Autodesk Inventor part; units mm, degrees
(part 4 of 5)
  line L786 (-10.0052, -6.7941) -> (-10.0052, -6.9319)
  line L787 (-10.0052, -6.9319) -> (-11.0441, -6.9319)
  spline S867 degree 2 poles (-11.0441, -6.9319) (-11.0441, -7.1928) (-10.7816, -7.47) (-10.5482, -7.47) knots 0 0 0 1 2 2 2
  spline S868 degree 2 poles (-10.5482, -7.47) (-10.4655, -7.47) (-10.3051, -7.4327) (-10.2402, -7.4035) knots 0 0 0 1 2 2 2
  spline S869 degree 2 poles (-10.2402, -7.4035) (-10.1722, -7.3711) (-10.0782, -7.3144) (-10.0474, -7.2884) knots 0 0 0 1 2 2 2
  line L788 (-10.0474, -7.2884) -> (-10.0328, -7.2884)
  line L789 (-10.0328, -7.2884) -> (-10.0328, -7.564)
  spline S870 degree 2 poles (-10.0328, -7.564) (-10.0765, -7.5818) (-10.2094, -7.6337) (-10.2613, -7.6482) knots 0 0 0 1 2 2 2
  spline S871 degree 2 poles (-10.2613, -7.6482) (-10.3342, -7.6693) (-10.4542, -7.6904) (-10.5449, -7.6904) knots 0 0 0 1 2 2 2
  spline S872 degree 2 poles (-10.2516, -6.739) (-10.2548, -6.6369) (-10.297, -6.4878) (-10.3375, -6.4376) knots 0 0 0 1 2 2 2
  spline S873 degree 2 poles (-10.3375, -6.4376) (-10.3812, -6.3808) (-10.519, -6.3209) (-10.6211, -6.3209) knots 0 0 0 1 2 2 2
  spline S874 degree 2 poles (-10.6211, -6.3209) (-10.7216, -6.3209) (-10.8626, -6.3808) (-10.921, -6.4392) knots 0 0 0 1 2 2 2
  spline S875 degree 2 poles (-10.921, -6.4392) (-10.9777, -6.4991) (-11.036, -6.6434) (-11.0441, -6.739) knots 0 0 0 1 2 2 2
  line L790 (-11.0441, -6.739) -> (-10.2516, -6.739)
  line L791 (-9.4915, -7.6564) -> (-9.7443, -7.6564)
  line L792 (-9.7443, -7.6564) -> (-9.7443, -5.5672)
  line L793 (-9.7443, -5.5672) -> (-9.4915, -5.5672)
  line L794 (-9.4915, -5.5672) -> (-9.4915, -7.6564)
  spline S876 degree 2 poles (-8.4688, -7.6904) (-8.8286, -7.6904) (-9.224, -7.2868) (-9.224, -6.914) knots 0 0 0 1 2 2 2
  spline S877 degree 2 poles (-9.224, -6.914) (-9.224, -6.5478) (-8.8399, -6.1134) (-8.5304, -6.1134) knots 0 0 0 1 2 2 2
  spline S878 degree 2 poles (-8.5304, -6.1134) (-8.391, -6.1134) (-8.1754, -6.1944) (-8.096, -6.2803) knots 0 0 0 1 2 2 2
  spline S879 degree 2 poles (-8.096, -6.2803) (-8.015, -6.3662) (-7.9291, -6.6142) (-7.9291, -6.7941) knots 0 0 0 1 2 2 2
  line L795 (-7.9291, -6.7941) -> (-7.9291, -6.9319)
  line L796 (-7.9291, -6.9319) -> (-8.968, -6.9319)
  spline S880 degree 2 poles (-8.968, -6.9319) (-8.968, -7.1928) (-8.7054, -7.47) (-8.472, -7.47) knots 0 0 0 1 2 2 2
  spline S881 degree 2 poles (-8.472, -7.47) (-8.3893, -7.47) (-8.2289, -7.4327) (-8.1641, -7.4035) knots 0 0 0 1 2 2 2
  spline S882 degree 2 poles (-8.1641, -7.4035) (-8.096, -7.3711) (-8.002, -7.3144) (-7.9712, -7.2884) knots 0 0 0 1 2 2 2
  line L797 (-7.9712, -7.2884) -> (-7.9566, -7.2884)
  line L798 (-7.9566, -7.2884) -> (-7.9566, -7.564)
  spline S883 degree 2 poles (-7.9566, -7.564) (-8.0004, -7.5818) (-8.1333, -7.6337) (-8.1851, -7.6482) knots 0 0 0 1 2 2 2
  spline S884 degree 2 poles (-8.1851, -7.6482) (-8.2581, -7.6693) (-8.378, -7.6904) (-8.4688, -7.6904) knots 0 0 0 1 2 2 2
  spline S885 degree 2 poles (-8.1754, -6.739) (-8.1787, -6.6369) (-8.2208, -6.4878) (-8.2613, -6.4376) knots 0 0 0 1 2 2 2
  spline S886 degree 2 poles (-8.2613, -6.4376) (-8.3051, -6.3808) (-8.4428, -6.3209) (-8.5449, -6.3209) knots 0 0 0 1 2 2 2
  spline S887 degree 2 poles (-8.5449, -6.3209) (-8.6454, -6.3209) (-8.7864, -6.3808) (-8.8448, -6.4392) knots 0 0 0 1 2 2 2
  spline S888 degree 2 poles (-8.8448, -6.4392) (-8.9015, -6.4991) (-8.9599, -6.6434) (-8.968, -6.739) knots 0 0 0 1 2 2 2
  line L799 (-8.968, -6.739) -> (-8.1754, -6.739)
  spline S889 degree 2 poles (-28.3034, -10.0611) (-28.3034, -10.2556) (-28.5822, -10.5328) (-28.7767, -10.5328) knots 0 0 0 1 2 2 2
  spline S890 degree 2 poles (-28.7767, -10.5328) (-28.9712, -10.5328) (-29.2483, -10.2556) (-29.2483, -10.0611) knots 0 0 0 1 2 2 2
  spline S891 degree 2 poles (-29.2483, -10.0611) (-29.2483, -9.8666) (-28.9712, -9.5895) (-28.7767, -9.5895) knots 0 0 0 1 2 2 2
  spline S892 degree 2 poles (-28.7767, -9.5895) (-28.5822, -9.5895) (-28.3034, -9.8666) (-28.3034, -10.0611) knots 0 0 0 1 2 2 2
  spline S893 degree 2 poles (-22.6406, -10.985) (-22.8577, -10.985) (-23.1624, -10.8942) (-23.297, -10.8294) knots 0 0 0 1 2 2 2
  line L800 (-23.297, -10.8294) -> (-23.297, -10.4955)
  line L801 (-23.297, -10.4955) -> (-23.2775, -10.4955)
  spline S894 degree 2 poles (-23.2775, -10.4955) (-23.1462, -10.6187) (-22.814, -10.7548) (-22.66, -10.7548) knots 0 0 0 1 2 2 2
  spline S895 degree 2 poles (-22.66, -10.7548) (-22.4396, -10.7548) (-22.2143, -10.5717) (-22.2143, -10.4209) knots 0 0 0 1 2 2 2
  spline S896 degree 2 poles (-22.2143, -10.4209) (-22.2143, -10.301) (-22.3326, -10.1519) (-22.4607, -10.1146) knots 0 0 0 1 2 2 2
  spline S897 degree 2 poles (-22.4607, -10.1146) (-22.553, -10.0887) (-22.707, -10.053) (-22.8221, -10.0239) knots 0 0 0 1 2 2 2
  spline S898 degree 2 poles (-22.8221, -10.0239) (-22.9258, -9.9963) (-23.0895, -9.9136) (-23.1527, -9.8472) knots 0 0 0 1 2 2 2
  spline S899 degree 2 poles (-23.1527, -9.8472) (-23.2143, -9.7807) (-23.2824, -9.6025) (-23.2824, -9.4858) knots 0 0 0 1 2 2 2
  spline S900 degree 2 poles (-23.2824, -9.4858) (-23.2824, -9.2427) (-22.9031, -8.9136) (-22.6098, -8.9136) knots 0 0 0 1 2 2 2
  spline S901 degree 2 poles (-22.6098, -8.9136) (-22.4412, -8.9136) (-22.143, -8.9801) (-22.015, -9.0433) knots 0 0 0 1 2 2 2
  line L802 (-22.015, -9.0433) -> (-22.015, -9.361)
  line L803 (-22.015, -9.361) -> (-22.0344, -9.361)
  spline S902 degree 2 poles (-22.0344, -9.361) (-22.13, -9.2734) (-22.4282, -9.1438) (-22.5919, -9.1438) knots 0 0 0 1 2 2 2
  spline S903 degree 2 poles (-22.5919, -9.1438) (-22.7767, -9.1438) (-23.0052, -9.3172) (-23.0052, -9.4582) knots 0 0 0 1 2 2 2
  spline S904 degree 2 poles (-23.0052, -9.4582) (-23.0052, -9.5846) (-22.8707, -9.7354) (-22.7443, -9.7694) knots 0 0 0 1 2 2 2
  spline S905 degree 2 poles (-22.7443, -9.7694) (-22.66, -9.7921) (-22.4153, -9.8504) (-22.3342, -9.8747) knots 0 0 0 1 2 2 2
  spline S906 degree 2 poles (-22.3342, -9.8747) (-22.1284, -9.938) (-21.9372, -10.1924) (-21.9372, -10.3788) knots 0 0 0 1 2 2 2
  spline S907 degree 2 poles (-21.9372, -10.3788) (-21.9372, -10.4971) (-22.0328, -10.724) (-22.1187, -10.8034) knots 0 0 0 1 2 2 2
  spline S908 degree 2 poles (-22.1187, -10.8034) (-22.2143, -10.891) (-22.4574, -10.985) (-22.6406, -10.985) knots 0 0 0 1 2 2 2
  spline S909 degree 2 poles (-20.4526, -10.1989) (-20.4526, -10.5781) (-20.8172, -10.9914) (-21.1219, -10.9914) knots 0 0 0 1 2 2 2
  spline S910 degree 2 poles (-21.1219, -10.9914) (-21.4347, -10.9914) (-21.7929, -10.5652) (-21.7929, -10.1989) knots 0 0 0 1 2 2 2
  spline S911 degree 2 poles (-21.7929, -10.1989) (-21.7929, -9.8229) (-21.4234, -9.4063) (-21.1219, -9.4063) knots 0 0 0 1 2 2 2
  spline S912 degree 2 poles (-21.1219, -9.4063) (-20.8172, -9.4063) (-20.4526, -9.8213) (-20.4526, -10.1989) knots 0 0 0 1 2 2 2
  spline S913 degree 2 poles (-20.7135, -10.1989) (-20.7135, -9.9072) (-20.9258, -9.6235) (-21.1219, -9.6235) knots 0 0 0 1 2 2 2
  spline S914 degree 2 poles (-21.1219, -9.6235) (-21.318, -9.6235) (-21.532, -9.9072) (-21.532, -10.1989) knots 0 0 0 1 2 2 2
  spline S915 degree 2 poles (-21.532, -10.1989) (-21.532, -10.4825) (-21.318, -10.7743) (-21.1219, -10.7743) knots 0 0 0 1 2 2 2
  spline S916 degree 2 poles (-21.1219, -10.7743) (-20.9274, -10.7743) (-20.7135, -10.4874) (-20.7135, -10.1989) knots 0 0 0 1 2 2 2
  spline S917 degree 2 poles (-19.5968, -10.9833) (-19.7524, -10.9833) (-20.0101, -10.8877) (-20.1025, -10.7905) knots 0 0 0 1 2 2 2
  spline S918 degree 2 poles (-20.1025, -10.7905) (-20.1949, -10.6948) (-20.297, -10.3999) (-20.297, -10.2021) knots 0 0 0 1 2 2 2
  spline S919 degree 2 poles (-20.297, -10.2021) (-20.297, -10.0044) (-20.1916, -9.7159) (-20.1025, -9.6187) knots 0 0 0 1 2 2 2
  spline S920 degree 2 poles (-20.1025, -9.6187) (-20.0133, -9.5198) (-19.7492, -9.4145) (-19.5968, -9.4145) knots 0 0 0 1 2 2 2
  spline S921 degree 2 poles (-19.5968, -9.4145) (-19.4736, -9.4145) (-19.2435, -9.4841) (-19.1543, -9.5295) knots 0 0 0 1 2 2 2
  line L804 (-19.1543, -9.5295) -> (-19.1543, -9.8132)
  line L805 (-19.1543, -9.8132) -> (-19.1689, -9.8132)
  spline S922 degree 2 poles (-19.1689, -9.8132) (-19.1965, -9.7905) (-19.2808, -9.7321) (-19.3407, -9.7013) knots 0 0 0 1 2 2 2
  spline S923 degree 2 poles (-19.3407, -9.7013) (-19.3942, -9.6754) (-19.5368, -9.6349) (-19.6017, -9.6349) knots 0 0 0 1 2 2 2
  spline S924 degree 2 poles (-19.6017, -9.6349) (-19.7978, -9.6349) (-20.036, -9.9315) (-20.036, -10.2021) knots 0 0 0 1 2 2 2
  spline S925 degree 2 poles (-20.036, -10.2021) (-20.036, -10.4663) (-19.8059, -10.7629) (-19.6017, -10.7629) knots 0 0 0 1 2 2 2
  spline S926 degree 2 poles (-19.6017, -10.7629) (-19.4785, -10.7629) (-19.2548, -10.6608) (-19.1689, -10.5814) knots 0 0 0 1 2 2 2
  line L806 (-19.1689, -10.5814) -> (-19.1543, -10.5814)
  line L807 (-19.1543, -10.5814) -> (-19.1543, -10.865)
  spline S927 degree 2 poles (-19.1543, -10.865) (-19.1916, -10.8828) (-19.3051, -10.9331) (-19.3505, -10.9444) knots 0 0 0 1 2 2 2
  spline S928 degree 2 poles (-19.3505, -10.9444) (-19.4153, -10.9639) (-19.5174, -10.9833) (-19.5968, -10.9833) knots 0 0 0 1 2 2 2
  spline S929 degree 2 poles (-18.3278, -10.9833) (-18.4834, -10.9833) (-18.7411, -10.8877) (-18.8334, -10.7905) knots 0 0 0 1 2 2 2
  spline S930 degree 2 poles (-18.8334, -10.7905) (-18.9258, -10.6948) (-19.0279, -10.3999) (-19.0279, -10.2021) knots 0 0 0 1 2 2 2
  spline S931 degree 2 poles (-19.0279, -10.2021) (-19.0279, -10.0044) (-18.9226, -9.7159) (-18.8334, -9.6187) knots 0 0 0 1 2 2 2
  spline S932 degree 2 poles (-18.8334, -9.6187) (-18.7443, -9.5198) (-18.4801, -9.4145) (-18.3278, -9.4145) knots 0 0 0 1 2 2 2
  spline S933 degree 2 poles (-18.3278, -9.4145) (-18.2046, -9.4145) (-17.9744, -9.4841) (-17.8853, -9.5295) knots 0 0 0 1 2 2 2
  line L808 (-17.8853, -9.5295) -> (-17.8853, -9.8132)
  line L809 (-17.8853, -9.8132) -> (-17.8999, -9.8132)
  spline S934 degree 2 poles (-17.8999, -9.8132) (-17.9274, -9.7905) (-18.0117, -9.7321) (-18.0717, -9.7013) knots 0 0 0 1 2 2 2
  spline S935 degree 2 poles (-18.0717, -9.7013) (-18.1252, -9.6754) (-18.2678, -9.6349) (-18.3326, -9.6349) knots 0 0 0 1 2 2 2
  spline S936 degree 2 poles (-18.3326, -9.6349) (-18.5287, -9.6349) (-18.767, -9.9315) (-18.767, -10.2021) knots 0 0 0 1 2 2 2
  spline S937 degree 2 poles (-18.767, -10.2021) (-18.767, -10.4663) (-18.5368, -10.7629) (-18.3326, -10.7629) knots 0 0 0 1 2 2 2
  spline S938 degree 2 poles (-18.3326, -10.7629) (-18.2094, -10.7629) (-17.9858, -10.6608) (-17.8999, -10.5814) knots 0 0 0 1 2 2 2
  line L810 (-17.8999, -10.5814) -> (-17.8853, -10.5814)
  line L811 (-17.8853, -10.5814) -> (-17.8853, -10.865)
  spline S939 degree 2 poles (-17.8853, -10.865) (-17.9226, -10.8828) (-18.036, -10.9331) (-18.0814, -10.9444) knots 0 0 0 1 2 2 2
  spline S940 degree 2 poles (-18.0814, -10.9444) (-18.1462, -10.9639) (-18.2483, -10.9833) (-18.3278, -10.9833) knots 0 0 0 1 2 2 2
  line L812 (-17.3975, -10.9493) -> (-17.6503, -10.9493)
  line L813 (-17.6503, -10.9493) -> (-17.6503, -9.4485)
  line L814 (-17.6503, -9.4485) -> (-17.3975, -9.4485)
  line L815 (-17.3975, -9.4485) -> (-17.3975, -10.9493)
  line L816 (-17.3796, -9.1989) -> (-17.6665, -9.1989)
  line L817 (-17.6665, -9.1989) -> (-17.6665, -8.9363)
  line L818 (-17.6665, -8.9363) -> (-17.3796, -8.9363)
  line L819 (-17.3796, -8.9363) -> (-17.3796, -9.1989)
  spline S941 degree 2 poles (-15.7929, -10.1989) (-15.7929, -10.5781) (-16.1576, -10.9914) (-16.4623, -10.9914) knots 0 0 0 1 2 2 2
  spline S942 degree 2 poles (-16.4623, -10.9914) (-16.7751, -10.9914) (-17.1333, -10.5652) (-17.1333, -10.1989) knots 0 0 0 1 2 2 2
  spline S943 degree 2 poles (-17.1333, -10.1989) (-17.1333, -9.8229) (-16.7637, -9.4063) (-16.4623, -9.4063) knots 0 0 0 1 2 2 2
  spline S944 degree 2 poles (-16.4623, -9.4063) (-16.1576, -9.4063) (-15.7929, -9.8213) (-15.7929, -10.1989) knots 0 0 0 1 2 2 2
  spline S945 degree 2 poles (-16.0539, -10.1989) (-16.0539, -9.9072) (-16.2662, -9.6235) (-16.4623, -9.6235) knots 0 0 0 1 2 2 2
  spline S946 degree 2 poles (-16.4623, -9.6235) (-16.6584, -9.6235) (-16.8723, -9.9072) (-16.8723, -10.1989) knots 0 0 0 1 2 2 2
  spline S947 degree 2 poles (-16.8723, -10.1989) (-16.8723, -10.4825) (-16.6584, -10.7743) (-16.4623, -10.7743) knots 0 0 0 1 2 2 2
  spline S948 degree 2 poles (-16.4623, -10.7743) (-16.2678, -10.7743) (-16.0539, -10.4874) (-16.0539, -10.1989) knots 0 0 0 1 2 2 2
  line L820 (-13.4963, -10.9493) -> (-14.6552, -10.9493)
  line L821 (-14.6552, -10.9493) -> (-14.6552, -8.9493)
  line L822 (-14.6552, -8.9493) -> (-14.3893, -8.9493)
  line L823 (-14.3893, -8.9493) -> (-14.3893, -10.7127)
  line L824 (-14.3893, -10.7127) -> (-13.4963, -10.7127)
  line L825 (-13.4963, -10.7127) -> (-13.4963, -10.9493)
  spline S949 degree 2 poles (-12.6552, -10.9833) (-13.015, -10.9833) (-13.4104, -10.5798) (-13.4104, -10.207) knots 0 0 0 1 2 2 2
  spline S950 degree 2 poles (-13.4104, -10.207) (-13.4104, -9.8407) (-13.0263, -9.4063) (-12.7167, -9.4063) knots 0 0 0 1 2 2 2
  spline S951 degree 2 poles (-12.7167, -9.4063) (-12.5774, -9.4063) (-12.3618, -9.4874) (-12.2824, -9.5733) knots 0 0 0 1 2 2 2
  spline S952 degree 2 poles (-12.2824, -9.5733) (-12.2013, -9.6592) (-12.1154, -9.9072) (-12.1154, -10.0871) knots 0 0 0 1 2 2 2
  line L826 (-12.1154, -10.0871) -> (-12.1154, -10.2248)
  line L827 (-12.1154, -10.2248) -> (-13.1543, -10.2248)
  spline S953 degree 2 poles (-13.1543, -10.2248) (-13.1543, -10.4858) (-12.8918, -10.7629) (-12.6584, -10.7629) knots 0 0 0 1 2 2 2
  spline S954 degree 2 poles (-12.6584, -10.7629) (-12.5757, -10.7629) (-12.4153, -10.7256) (-12.3505, -10.6965) knots 0 0 0 1 2 2 2
  spline S955 degree 2 poles (-12.3505, -10.6965) (-12.2824, -10.664) (-12.1884, -10.6073) (-12.1576, -10.5814) knots 0 0 0 1 2 2 2
  line L828 (-12.1576, -10.5814) -> (-12.143, -10.5814)
  line L829 (-12.143, -10.5814) -> (-12.143, -10.8569)
  spline S956 degree 2 poles (-12.143, -10.8569) (-12.1868, -10.8747) (-12.3197, -10.9266) (-12.3715, -10.9412) knots 0 0 0 1 2 2 2
  spline S957 degree 2 poles (-12.3715, -10.9412) (-12.4445, -10.9623) (-12.5644, -10.9833) (-12.6552, -10.9833) knots 0 0 0 1 2 2 2
  spline S958 degree 2 poles (-12.3618, -10.032) (-12.365, -9.9298) (-12.4072, -9.7807) (-12.4477, -9.7305) knots 0 0 0 1 2 2 2
  spline S959 degree 2 poles (-12.4477, -9.7305) (-12.4915, -9.6738) (-12.6292, -9.6138) (-12.7313, -9.6138) knots 0 0 0 1 2 2 2
  spline S960 degree 2 poles (-12.7313, -9.6138) (-12.8318, -9.6138) (-12.9728, -9.6738) (-13.0312, -9.7321) knots 0 0 0 1 2 2 2
  spline S961 degree 2 poles (-13.0312, -9.7321) (-13.0879, -9.7921) (-13.1462, -9.9363) (-13.1543, -10.032) knots 0 0 0 1 2 2 2
  line L830 (-13.1543, -10.032) -> (-12.3618, -10.032)
  spline S962 degree 2 poles (-10.626, -10.1989) (-10.626, -10.5781) (-10.9906, -10.9914) (-11.2953, -10.9914) knots 0 0 0 1 2 2 2
  spline S963 degree 2 poles (-11.2953, -10.9914) (-11.6081, -10.9914) (-11.9663, -10.5652) (-11.9663, -10.1989) knots 0 0 0 1 2 2 2
  spline S964 degree 2 poles (-11.9663, -10.1989) (-11.9663, -9.8229) (-11.5968, -9.4063) (-11.2953, -9.4063) knots 0 0 0 1 2 2 2
  spline S965 degree 2 poles (-11.2953, -9.4063) (-10.9906, -9.4063) (-10.626, -9.8213) (-10.626, -10.1989) knots 0 0 0 1 2 2 2
  spline S966 degree 2 poles (-10.8869, -10.1989) (-10.8869, -9.9072) (-11.0992, -9.6235) (-11.2953, -9.6235) knots 0 0 0 1 2 2 2
  spline S967 degree 2 poles (-11.2953, -9.6235) (-11.4915, -9.6235) (-11.7054, -9.9072) (-11.7054, -10.1989) knots 0 0 0 1 2 2 2
  spline S968 degree 2 poles (-11.7054, -10.1989) (-11.7054, -10.4825) (-11.4915, -10.7743) (-11.2953, -10.7743) knots 0 0 0 1 2 2 2
  spline S969 degree 2 poles (-11.2953, -10.7743) (-11.1009, -10.7743) (-10.8869, -10.4874) (-10.8869, -10.1989) knots 0 0 0 1 2 2 2
  line L831 (-9.1884, -10.9493) -> (-9.4412, -10.9493)
  line L832 (-9.4412, -10.9493) -> (-9.4412, -10.0935)
  spline S970 degree 2 poles (-9.4412, -10.0935) (-9.4412, -9.9898) (-9.4607, -9.8115) (-9.4898, -9.758) knots 0 0 0 1 2 2 2
  spline S971 degree 2 poles (-9.4898, -9.758) (-9.5206, -9.7013) (-9.6308, -9.6462) (-9.7248, -9.6462) knots 0 0 0 1 2 2 2
  spline S972 degree 2 poles (-9.7248, -9.6462) (-9.8188, -9.6462) (-10.0182, -9.7467) (-10.1138, -9.8277) knots 0 0 0 1 2 2 2
  line L833 (-10.1138, -9.8277) -> (-10.1138, -10.9493)
  line L834 (-10.1138, -10.9493) -> (-10.3667, -10.9493)
  line L835 (-10.3667, -10.9493) -> (-10.3667, -9.4485)
  line L836 (-10.3667, -9.4485) -> (-10.1138, -9.4485)
  line L837 (-10.1138, -9.4485) -> (-10.1138, -9.6154)
  spline S973 degree 2 poles (-10.1138, -9.6154) (-10.0004, -9.5133) (-9.7816, -9.4063) (-9.6584, -9.4063) knots 0 0 0 1 2 2 2
  spline S974 degree 2 poles (-9.6584, -9.4063) (-9.438, -9.4063) (-9.1884, -9.6981) (-9.1884, -9.9752) knots 0 0 0 1 2 2 2
  line L838 (-9.1884, -9.9752) -> (-9.1884, -10.9493)
  spline S975 degree 2 poles (-7.9971, -10.7905) (-8.0279, -10.8132) (-8.1317, -10.8942) (-8.1803, -10.9185) knots 0 0 0 1 2 2 2
  spline S976 degree 2 poles (-8.1803, -10.9185) (-8.2467, -10.9542) (-8.3715, -10.9914) (-8.485, -10.9914) knots 0 0 0 1 2 2 2
  spline S977 degree 2 poles (-8.485, -10.9914) (-8.5774, -10.9914) (-8.7443, -10.9217) (-8.8075, -10.8585) knots 0 0 0 1 2 2 2
  spline S978 degree 2 poles (-8.8075, -10.8585) (-8.8675, -10.7969) (-8.9404, -10.6154) (-8.9404, -10.5149) knots 0 0 0 1 2 2 2
  spline S979 degree 2 poles (-8.9404, -10.5149) (-8.9404, -10.3593) (-8.8091, -10.1389) (-8.6665, -10.0757) knots 0 0 0 1 2 2 2
  spline S980 degree 2 poles (-8.6665, -10.0757) (-8.5401, -10.0174) (-8.1965, -9.9736) (-7.9971, -9.9623) knots 0 0 0 1 2 2 2
  line L839 (-7.9971, -9.9623) -> (-7.9971, -9.9136)
  spline S981 degree 2 poles (-7.9971, -9.9136) (-7.9971, -9.8261) (-8.0506, -9.7175) (-8.0992, -9.6867) knots 0 0 0 1 2 2 2
  spline S982 degree 2 poles (-8.0992, -9.6867) (-8.1479, -9.6559) (-8.2872, -9.6365) (-8.3618, -9.6365) knots 0 0 0 1 2 2 2
  spline S983 degree 2 poles (-8.3618, -9.6365) (-8.4493, -9.6365) (-8.6859, -9.6884) (-8.8043, -9.7386) knots 0 0 0 1 2 2 2
  line L840 (-8.8043, -9.7386) -> (-8.8188, -9.7386)
  line L841 (-8.8188, -9.7386) -> (-8.8188, -9.4809)
  spline S984 degree 2 poles (-8.8188, -9.4809) (-8.7492, -9.4615) (-8.4882, -9.4128) (-8.3602, -9.4128) knots 0 0 0 1 2 2 2
  spline S985 degree 2 poles (-8.3602, -9.4128) (-8.2046, -9.4128) (-7.9923, -9.4615) (-7.908, -9.5247) knots 0 0 0 1 2 2 2
  spline S986 degree 2 poles (-7.908, -9.5247) (-7.8253, -9.5863) (-7.7443, -9.7824) (-7.7443, -9.9234) knots 0 0 0 1 2 2 2
  line L842 (-7.7443, -9.9234) -> (-7.7443, -10.9493)
  line L843 (-7.7443, -10.9493) -> (-7.9971, -10.9493)
  line L844 (-7.9971, -10.9493) -> (-7.9971, -10.7905)
  line L845 (-7.9971, -10.5798) -> (-7.9971, -10.1632)
  spline S987 degree 2 poles (-7.9971, -10.1632) (-8.0879, -10.1713) (-8.3618, -10.1989) (-8.4477, -10.2248) knots 0 0 0 1 2 2 2
  spline S988 degree 2 poles (-8.4477, -10.2248) (-8.5482, -10.2556) (-8.6795, -10.3837) (-8.6795, -10.4971) knots 0 0 0 1 2 2 2
  spline S989 degree 2 poles (-8.6795, -10.4971) (-8.6795, -10.6268) (-8.5336, -10.758) (-8.3942, -10.758) knots 0 0 0 1 2 2 2
  spline S990 degree 2 poles (-8.3942, -10.758) (-8.2759, -10.758) (-8.0814, -10.6559) (-7.9971, -10.5798) knots 0 0 0 1 2 2 2
  line L846 (-6.5936, -9.7192) -> (-6.6065, -9.7192)
  spline S991 degree 2 poles (-6.6065, -9.7192) (-6.6357, -9.711) (-6.6989, -9.7078) (-6.7427, -9.7078) knots 0 0 0 1 2 2 2
  spline S992 degree 2 poles (-6.7427, -9.7078) (-6.8448, -9.7078) (-7.0458, -9.7969) (-7.1365, -9.8845) knots 0 0 0 1 2 2 2
  line L847 (-7.1365, -9.8845) -> (-7.1365, -10.9493)
  line L848 (-7.1365, -10.9493) -> (-7.3893, -10.9493)
  line L849 (-7.3893, -10.9493) -> (-7.3893, -9.4485)
  line L850 (-7.3893, -9.4485) -> (-7.1365, -9.4485)
  line L851 (-7.1365, -9.4485) -> (-7.1365, -9.6722)
  spline S993 degree 2 poles (-7.1365, -9.6722) (-6.9987, -9.549) (-6.7929, -9.4485) (-6.6957, -9.4485) knots 0 0 0 1 2 2 2
  spline S994 degree 2 poles (-6.6957, -9.4485) (-6.6568, -9.4485) (-6.6179, -9.4517) (-6.5936, -9.4566) knots 0 0 0 1 2 2 2
  line L852 (-6.5936, -9.4566) -> (-6.5936, -9.7192)
  line L853 (-5.2435, -10.9493) -> (-5.4963, -10.9493)
  line L854 (-5.4963, -10.9493) -> (-5.4963, -10.7969)
  spline S995 degree 2 poles (-5.4963, -10.7969) (-5.5547, -10.8456) (-5.6406, -10.9104) (-5.6989, -10.938) knots 0 0 0 1 2 2 2
  spline S996 degree 2 poles (-5.6989, -10.938) (-5.7524, -10.9639) (-5.8675, -10.9914) (-5.9436, -10.9914) knots 0 0 0 1 2 2 2
  spline S997 degree 2 poles (-5.9436, -10.9914) (-6.0668, -10.9914) (-6.2743, -10.8893) (-6.3472, -10.7905) knots 0 0 0 1 2 2 2
  spline S998 degree 2 poles (-6.3472, -10.7905) (-6.4201, -10.6916) (-6.5012, -10.3999) (-6.5012, -10.2102) knots 0 0 0 1 2 2 2
  spline S999 degree 2 poles (-6.5012, -10.2102) (-6.5012, -10.0125) (-6.3991, -9.724) (-6.3099, -9.6154) knots 0 0 0 1 2 2 2
  spline S1000 degree 2 poles (-6.3099, -9.6154) (-6.2273, -9.5182) (-5.9955, -9.4063) (-5.8675, -9.4063) knots 0 0 0 1 2 2 2
  spline S1001 degree 2 poles (-5.8675, -9.4063) (-5.7556, -9.4063) (-5.5887, -9.4566) (-5.4963, -9.5085) knots 0 0 0 1 2 2 2
  line L855 (-5.4963, -9.5085) -> (-5.4963, -8.8602)
  line L856 (-5.4963, -8.8602) -> (-5.2435, -8.8602)
  line L857 (-5.2435, -8.8602) -> (-5.2435, -10.9493)
  line L858 (-5.4963, -10.5846) -> (-5.4963, -9.7175)
  spline S1002 degree 2 poles (-5.4963, -9.7175) (-5.5903, -9.6722) (-5.7394, -9.6381) (-5.8253, -9.6381) knots 0 0 0 1 2 2 2
  spline S1003 degree 2 poles (-5.8253, -9.6381) (-6.0198, -9.6381) (-6.2402, -9.9298) (-6.2402, -10.2054) knots 0 0 0 1 2 2 2
  spline S1004 degree 2 poles (-6.2402, -10.2054) (-6.2402, -10.4712) (-6.0717, -10.7516) (-5.8853, -10.7516) knots 0 0 0 1 2 2 2
  spline S1005 degree 2 poles (-5.8853, -10.7516) (-5.7864, -10.7516) (-5.5855, -10.6608) (-5.4963, -10.5846) knots 0 0 0 1 2 2 2
  spline S1006 degree 2 poles (-3.6438, -10.1989) (-3.6438, -10.5781) (-4.0085, -10.9914) (-4.3132, -10.9914) knots 0 0 0 1 2 2 2
  spline S1007 degree 2 poles (-4.3132, -10.9914) (-4.626, -10.9914) (-4.9842, -10.5652) (-4.9842, -10.1989) knots 0 0 0 1 2 2 2
  spline S1008 degree 2 poles (-4.9842, -10.1989) (-4.9842, -9.8229) (-4.6146, -9.4063) (-4.3132, -9.4063) knots 0 0 0 1 2 2 2
  spline S1009 degree 2 poles (-4.3132, -9.4063) (-4.0085, -9.4063) (-3.6438, -9.8213) (-3.6438, -10.1989) knots 0 0 0 1 2 2 2
  spline S1010 degree 2 poles (-3.9047, -10.1989) (-3.9047, -9.9072) (-4.1171, -9.6235) (-4.3132, -9.6235) knots 0 0 0 1 2 2 2
  spline S1011 degree 2 poles (-4.3132, -9.6235) (-4.5093, -9.6235) (-4.7232, -9.9072) (-4.7232, -10.1989) knots 0 0 0 1 2 2 2
  spline S1012 degree 2 poles (-4.7232, -10.1989) (-4.7232, -10.4825) (-4.5093, -10.7743) (-4.3132, -10.7743) knots 0 0 0 1 2 2 2
  spline S1013 degree 2 poles (-4.3132, -10.7743) (-4.1187, -10.7743) (-3.9047, -10.4874) (-3.9047, -10.1989) knots 0 0 0 1 2 2 2
  point P0 (0, 0)
  constraints: 48 end point, 12 horizontal, 12 vertical, 26 other
extrude "Estrusione2" cut sketch "Schizzo2" against normal blind 1 contours S0 S1 L32 L33 L34 L35 L36 S2 S3 | L40 S8 S9 L41 L42 L43 L44 L45 S10 S11 L46 | S12 S13 S14 S15 | S20 S21 S22 S23 L47 S24 S25 S26 S27 S28 L48 L49 L50 S29 S30 L51 L52 | S35 S36 S37 S38 L54 L55 S39 S40 S41 L56 L57 S42 S43 | S48 L59 L60 L61 L62 L63 L64 L65 L66 L67 L68 L69 S49 S50 S51 L70 L71 S52 | S53 L72 L73 L74 L75 L76 L77 L78 L79 L80 L81 L82 S54 S55 S56 L83 L84 S57 | S58 S59 S60 S61 | L85 L86 S66 S67 S68 S69 S70 S71 S72 L87 L88 L89 | L91 L92 L93 L94 | L95 L96 L97 L98 | L99 S77 S78 S79 S80 L100 L101 L102 S81 S82 S83 L103 L104 L105 L106 L107 S84 S85 S86 S87 S88 L108 L109 | S89 S90 S91 S92 L110 L111 S93 S94 S95 L112 L113 S96 S97 | S102 S103 S104 S105 S106 L115 L116 S107 S108 S109 S110 S111 L117 L118 S112 S113 | S114 S115 S116 S117 S118 L119 L120 S119 S120 S121 S122 S123 L121 L122 S124 S125 | S126 S127 S128 S129 S130 S131 L123 S132 S133 S134 L124 L125 S135 S136 S137 L126 L127 L128 | L130 L131 S142 S143 S144 L132 L133 L134 L135 L136 S145 S146 L137 | L138 L139 L140 L141 | L142 L143 L144 L145 | S147 S148 S149 S150 S151 L146 L147 S152 S153 S154 S155 S156 L148 L149 S157 S158 | S159 S160 S161 S162 S163 S164 L150 S165 S166 S167 L151 L152 S168 S169 S170 L153 L154 L155 | L157 L158 S175 S176 S177 S178 S179 S180 S181 L159 L160 L161 | S186 S187 S188 S189 L163 L164 S190 S191 S192 L165 L166 S193 S194 | L168 L169 L170 L171 | L172 L173 L174 L175 | S199 S200 S201 S202 L176 L177 S203 S204 S205 L178 L179 S206 S207 | L181 L182 L183 L184 L185 L186 L187 | L188 L189 L190 L191 | L192 L193 L194 L195 | S212 S213 L196 L197 L198 L199 L200 S214 S215 | L202 S220 S221 L203 L204 L205 L206 L207 S222 S223 L208 | S224 S225 S226 S227 S228 S229 L209 S230 S231 S232 L210 L211 S233 S234 S235 L212 L213 L214 | L216 L217 L218 L219 L220 L221 L222 L223 L224 L225 | L226 L227 L228 L229 | L230 L231 L232 L233 | S240 S241 S242 S243 | L234 L235 S248 S249 S250 L236 L237 L238 L239 L240 S251 S252 L241 | L242 L243 L244 L245 | L246 L247 L248 L249 | L250 L251 S253 S254 S255 S256 S257 S258 L252 L253 S259 S260 S261 S262 S263 L254 L255 | S264 S265 S266 S267 | L256 L257 L258 L259 L260 L261 S276 L262 L263 L264 L265 | S277 S278 S279 S280 S281 S282 S283 L266 L267 S284 S285 S286 S287 S288 | L268 L269 L270 L271 | L272 L273 S296 S297 S298 S299 S300 S301 L274 L275 S302 S303 S304 S305 S306 L276 L277 | S307 S308 S309 S310 | S319 S320 L278 L279 L280 S321 S322 S323 L281 S324 | S333 S334 S335 S336 S337 S338 L288 S339 S340 S341 L289 L290 S342 S343 S344 L291 L292 L293 | L295 L296 S349 S350 S351 L297 L298 L299 L300 L301 S352 S353 L302 | S354 S355 S356 S357 S358 L303 L304 S359 S360 S361 S362 S363 L305 L306 S364 S365 | S366 S367 S368 S369 | L307 L308 S374 S375 S376 S377 S378 S379 S380 L309 L310 L311 | L313 L314 L315 L316 | L317 L318 L319 L320 | S385 S386 L321 L322 L323 L324 L325 S387 S388 | L327 S393 S394 L328 L329 L330 L331 L332 S395 S396 L333 | S397 S398 S399 S400 | L334 L335 L336 L337 L338 L339 L340 | S405 S406 S407 S408 S409 S410 L341 S411 S412 S413 L342 L343 S414 S415 S416 L344 L345 L346 | S421 S422 L348 L349 L350 L351 L352 S423 S424 | S429 S430 S431 S432 L354 L355 S433 S434 S435 L356 L357 S436 S437 | L359 S442 S443 L360 L361 L362 L363 L364 S444 S445 L365 | L366 S446 S447 S448 S449 L367 L368 L369 S450 S451 S452 L370 L371 L372 L373 L374 S453 S454 S455 S456 S457 L375 L376 | S458 S459 S460 S461 | S466 L377 L378 L379 L380 L381 L382 L383 L384 L385 L386 L387 S467 S468 S469 L388 L389 S470 | S471 S472 S473 S474 | L390 S479 S480 L391 L392 L393 L394 L395 S481 S482 L396 | S483 S484 S485 S486 L397 L398 S487 S488 S489 L399 L400 S490 S491 | S496 S497 L402 L403 L404 S498 S499 | S504 S505 S506 S507 S508 S509 L408 L409 S510 S511 S512 S513 S514 S515 S516 S517 L410 L411 S518 S519 | L412 L413 L414 L415 L416 L417 L418 L419 | S520 S521 S522 S523 S524 L423 L424 S525 S526 S527 S528 S529 L425 L426 S530 S531 | L427 L428 S532 S533 S534 L429 L430 L431 S535 S536 S537 L432 L433 L434 | L435 S538 S539 L436 L437 L438 L439 L440 S540 S541 L441 | S542 S543 S544 S545 S546 S547 L442 S548 S549 S550 L443 L444 S551 S552 S553 L445 L446 L447 | L449 L450 S558 S559 S560 S561 S562 S563 S564 L451 L452 L453 | L455 L456 L457 L458 | L459 L460 L461 L462 | L463 L464 L465 L466 | L467 L468 L469 L470 | S569 S570 S571 S572 | L471 L472 L473 L474 L475 L476 L477 L478 | L482 L483 L484 L485 | L486 S573 S574 L487 L488 L489 L490 L491 L492 L493 L494 L495 L496 L497 S575 S576 L498 | S577 S578 S579 S580 S581 S582 L499 S583 S584 S585 L500 L501 S586 S587 S588 L502 L503 L504 | L506 L507 S593 S594 S595 L508 L509 L510 L511 L512 S596 S597 L513 | S598 S599 S600 S601 | L514 L515 L516 L517 L518 L519 L520 L521 L522 L523 L524 L525 | L526 S606 S607 S608 S609 L527 L528 L529 S610 S611 S612 L530 L531 L532 L533 L534 S613 S614 S615 S616 S617 L535 L536 | S618 S619 S620 S621 S622 S623 L537 S624 S625 S626 L538 L539 S627 S628 S629 L540 L541 L542 | L544 L545 S634 S635 S636 L546 L547 L548 L549 L550 S637 S638 L551 | L552 L553 S639 S640 S641 L554 L555 L556 S642 S643 S644 L557 L558 L559 | S645 S646 S647 S648 L560 L561 S649 S650 S651 L562 L563 S652 S653 | L565 L566 L567 L568 | S658 S659 S660 S661 L569 L570 S662 S663 S664 L571 L572 S665 S666 | S671 S672 S673 S674 | S675 S676 L574 L575 L576 S677 S678 S679 L577 S680 | S689 S690 S691 S692 S693 S694 L584 S695 S696 S697 L585 L586 S698 S699 S700 L587 L588 L589 | L591 L592 S705 S706 S707 S708 S709 S710 S711 L593 L594 L595 | S716 S717 S718 S719 S720 S721 L597 S722 S723 S724 L598 L599 S725 S726 S727 L600 L601 L602 | L604 L605 L606 L607 | S732 S733 S734 S735 S736 S737 L608 S738 S739 S740 L609 L610 S741 S742 S743 L611 L612 L613 | L615 S748 S749 S750 S751 L616 L617 L618 S752 S753 S754 L619 L620 L621 L622 L623 S755 S756 S757 S758 S759 L624 L625 | S760 S761 S762 S763 L626 L627 S764 S765 S766 L628 L629 S767 S768 | L631 L632 S773 S774 S775 L633 L634 L635 L636 L637 S776 S777 L638 | S778 L639 L640 L641 L642 L643 L644 L645 L646 L647 L648 L649 S779 S780 S781 L650 L651 S782 | L652 L653 L654 L655 | L656 L657 L658 L659 | L660 L661 L662 L663 L664 L665 L666 L667 L668 L669 | L670 L671 L672 L673 | L674 L675 L676 L677 | L678 L679 L680 L681 | L682 L683 L684 L685 | L686 L687 L688 L689 | S783 S784 L690 L691 L692 L693 L694 S785 S786 | S791 S792 L696 L697 L698 L699 L700 S793 S794 | S799 S800 S801 S802 | S807 S808 S809 S810 | L702 L703 L704 L705 L706 L707 L708 | L709 L710 L711 L712 | L713 L714 L715 L716 | S811 L717 L718 L719 L720 L721 L722 L723 L724 L725 L726 L727 S812 S813 S814 L728 L729 S815 | S816 L730 L731 L732 L733 L734 L735 L736 L737 L738 L739 L740 S817 S818 S819 L741 L742 S820 | L743 L744 L745 L746 | L747 L748 L749 L750 | S821 S822 S823 S824 S825 S826 L751 L752 S827 S828 S829 S830 S831 S832 L753 L754 L755 L756 L757 S833 S834 | S835 S836 S837 S838 S839 S840 L758 S841 S842 S843 L759 L760 S844 S845 S846 L761 L762 L763 | S851 S852 L765 L766 L767 L768 L769 S853 S854 | L771 S859 S860 L772 L773 L774 L775 L776 S861 S862 L777 | L778 L779 L780 L781 | L782 L783 L784 L785 | S863 S864 S865 S866 L786 L787 S867 S868 S869 L788 L789 S870 S871 | L791 L792 L793 L794 | S876 S877 S878 S879 L795 L796 S880 S881 S882 L797 L798 S883 S884 | S889 S890 S891 S892 | S893 L800 L801 S894 S895 S896 S897 S898 S899 S900 S901 L802 L803 S902 S903 S904 S905 S906 S907 S908 | S909 S910 S911 S912 | S917 S918 S919 S920 S921 L804 L805 S922 S923 S924 S925 S926 L806 L807 S927 S928 | S929 S930 S931 S932 S933 L808 L809 S934 S935 S936 S937 S938 L810 L811 S939 S940 | L812 L813 L814 L815 | L816 L817 L818 L819 | S941 S942 S943 S944 | L820 L821 L822 L823 L824 L825 | S949 S950 S951 S952 L826 L827 S953 S954 S955 L828 L829 S956 S957 | S962 S963 S964 S965 | L831 L832 S970 S971 S972 L833 L834 L835 L836 L837 S973 S974 L838 | S975 S976 S977 S978 S979 S980 L839 S981 S982 S983 L840 L841 S984 S985 S986 L842 L843 L844 | L846 S991 S992 L847 L848 L849 L850 L851 S993 S994 L852 | L853 L854 S995 S996 S997 S998 S999 S1000 S1001 L855 L856 L857 | S1006 S1007 S1008 S1009
sketch "Schizzo3" plane through (0, 0, 4) normal (0, 0, 1) x (1, 0, 0)
  line L0 (-31, -5) -> (-35, -5)
  line L1 (-35, -5) -> (-35, 0)
  line L2 (-35, 0) -> (-31, 0)
  line L3 (-31, 0) -> (-31, -5)
  line L4 (-35, 10) -> (-31, 10)
  line L5 (-31, 10) -> (-31, 5)
  line L6 (-31, 5) -> (-35, 5)
  line L7 (-35, 5) -> (-35, 10)
  line L8 (-31, -15) -> (-35, -15)
  line L9 (-35, -15) -> (-35, -10)
  line L10 (-35, -10) -> (-31, -10)
  line L11 (-31, -10) -> (-31, -15)
  line L12 (35, -5) -> (31, -5)
  line L13 (31, -5) -> (31, 0)
  line L14 (31, 0) -> (35, 0)
  line L15 (35, 0) -> (35, -5)
  line L16 (31, 10) -> (35, 10)
  line L17 (35, 10) -> (35, 5)
  line L18 (35, 5) -> (31, 5)
  line L19 (31, 5) -> (31, 10)
  line L20 (35, -15) -> (31, -15)
  line L21 (31, -15) -> (31, -10)
  line L22 (31, -10) -> (35, -10)
  line L23 (35, -10) -> (35, -15)
  point P0 (0, 0)
  constraints: 48 end point, 12 horizontal, 12 vertical, 24 other
extrude "Estrusione3" cut sketch "Schizzo3" against normal blind 10
sketch "Schizzo4" plane through (0, 0, 4) normal (0, 0, 1) x (1, 0, 0)
  line L0 (-31, 5) -> (-31, 10)
  line L1 (-31, 10) -> (-35, 10)
  line L2 (-35, 10) -> (-35, 12)
  arc A0 (-32, 15) -> (-35, 12) centre (-32, 12) ccw
  line L3 (-32, 15) -> (32, 15)
  arc A1 (35, 12) -> (32, 15) centre (32, 12) ccw
  line L4 (35, 12) -> (35, 10)
  line L5 (35, 10) -> (31, 10)
  line L6 (31, 10) -> (31, 5)
  line L7 (31, 5) -> (35, 5)
  line L8 (35, 5) -> (35, 0)
  line L9 (35, 0) -> (31, 0)
  line L10 (31, 0) -> (31, -5)
  line L11 (31, -5) -> (35, -5)
  line L12 (35, -5) -> (35, -10)
  line L13 (35, -10) -> (31, -10)
  line L14 (31, -10) -> (31, -15)
  line L15 (31, -15) -> (-31, -15)
  line L16 (-31, -15) -> (-31, -10)
  line L17 (-31, -10) -> (-35, -10)
  line L18 (-35, -10) -> (-35, -5)
  line L19 (-35, -5) -> (-31, -5)
  line L20 (-31, -5) -> (-31, 0)
  line L21 (-31, 0) -> (-35, 0)
  line L22 (-35, 0) -> (-35, 5)
  line L23 (-35, 5) -> (-31, 5)
  line L24 (-5.4963, -9.7175) -> (-5.4963, -10.5846)
  line L25 (-5.2435, -10.9493) -> (-5.2435, -8.8602)
  line L26 (-5.2435, -8.8602) -> (-5.4963, -8.8602)
  line L27 (-5.4963, -8.8602) -> (-5.4963, -9.5085)
  line L28 (-5.4963, -10.7969) -> (-5.4963, -10.9493)
  line L29 (-5.4963, -10.9493) -> (-5.2435, -10.9493)
  line L30 (-9.1884, -10.9493) -> (-9.1884, -9.9752)
  line L31 (-10.1138, -9.6154) -> (-10.1138, -9.4485)
  line L32 (-10.1138, -9.4485) -> (-10.3667, -9.4485)
  line L33 (-10.3667, -9.4485) -> (-10.3667, -10.9493)
  line L34 (-10.3667, -10.9493) -> (-10.1138, -10.9493)
  line L35 (-10.1138, -10.9493) -> (-10.1138, -9.8277)
  line L36 (-9.4412, -10.0935) -> (-9.4412, -10.9493)
  line L37 (-9.4412, -10.9493) -> (-9.1884, -10.9493)
  line L38 (-12.3618, -10.032) -> (-13.1543, -10.032)
  line L39 (-12.143, -10.8569) -> (-12.143, -10.5814)
  line L40 (-12.143, -10.5814) -> (-12.1576, -10.5814)
  line L41 (-13.1543, -10.2248) -> (-12.1154, -10.2248)
  line L42 (-12.1154, -10.2248) -> (-12.1154, -10.0871)
  line L43 (-17.3796, -9.1989) -> (-17.3796, -8.9363)
  line L44 (-17.3796, -8.9363) -> (-17.6665, -8.9363)
  line L45 (-17.6665, -8.9363) -> (-17.6665, -9.1989)
  line L46 (-17.6665, -9.1989) -> (-17.3796, -9.1989)
  line L47 (-17.8853, -10.865) -> (-17.8853, -10.5814)
  line L48 (-17.8853, -10.5814) -> (-17.8999, -10.5814)
  line L49 (-17.8999, -9.8132) -> (-17.8853, -9.8132)
  line L50 (-17.8853, -9.8132) -> (-17.8853, -9.5295)
  line L51 (-22.0344, -9.361) -> (-22.015, -9.361)
  line L52 (-22.015, -9.361) -> (-22.015, -9.0433)
  line L53 (-23.2775, -10.4955) -> (-23.297, -10.4955)
  line L54 (-23.297, -10.4955) -> (-23.297, -10.8294)
  line L55 (-9.4915, -7.6564) -> (-9.4915, -5.5672)
  line L56 (-9.4915, -5.5672) -> (-9.7443, -5.5672)
  line L57 (-9.7443, -5.5672) -> (-9.7443, -7.6564)
  line L58 (-9.7443, -7.6564) -> (-9.4915, -7.6564)
  line L59 (-10.2516, -6.739) -> (-11.0441, -6.739)
  line L60 (-10.0328, -7.564) -> (-10.0328, -7.2884)
  line L61 (-10.0328, -7.2884) -> (-10.0474, -7.2884)
  line L62 (-11.0441, -6.9319) -> (-10.0052, -6.9319)
  line L63 (-10.0052, -6.9319) -> (-10.0052, -6.7941)
  line L64 (-11.5676, -7.6564) -> (-11.5676, -6.1555)
  line L65 (-11.5676, -6.1555) -> (-11.8205, -6.1555)
  line L66 (-11.8205, -6.1555) -> (-11.8205, -7.6564)
  line L67 (-11.8205, -7.6564) -> (-11.5676, -7.6564)
  line L68 (-16.096, -7.5234) -> (-16.096, -6.6499)
  line L69 (-16.096, -6.6499) -> (-16.8221, -6.6499)
  line L70 (-16.8221, -6.6499) -> (-16.8221, -6.8833)
  line L71 (-16.8221, -6.8833) -> (-16.3586, -6.8833)
  line L72 (-16.3586, -6.8833) -> (-16.3586, -7.4003)
  line L73 (-16.1268, -6.1134) -> (-16.1041, -6.1134)
  line L74 (-16.1041, -6.1134) -> (-16.1041, -5.7925)
  line L75 (-18.848, -7.6564) -> (-18.848, -6.1555)
  line L76 (-18.848, -6.1555) -> (-19.1009, -6.1555)
  line L77 (-19.1009, -6.1555) -> (-19.1009, -7.6564)
  line L78 (-19.1009, -7.6564) -> (-18.848, -7.6564)
  line L79 (-20.2127, -7.6434) -> (-20.2127, -7.4165)
  line L80 (-20.2127, -7.4165) -> (-20.2273, -7.4165)
  line L81 (-20.6778, -7.0794) -> (-20.6778, -6.3646)
  line L82 (-20.6778, -6.3646) -> (-20.2127, -6.3646)
  line L83 (-20.2127, -6.3646) -> (-20.2127, -6.1555)
  line L84 (-20.2127, -6.1555) -> (-20.6778, -6.1555)
  line L85 (-20.6778, -6.1555) -> (-20.6778, -5.7244)
  line L86 (-20.6778, -5.7244) -> (-20.9307, -5.7244)
  line L87 (-20.9307, -5.7244) -> (-20.9307, -6.1555)
  line L88 (-20.9307, -6.1555) -> (-21.1009, -6.1555)
  line L89 (-21.1009, -6.1555) -> (-21.1009, -6.3646)
  line L90 (-21.1009, -6.3646) -> (-20.9307, -6.3646)
  line L91 (-20.9307, -6.3646) -> (-20.9307, -7.1961)
  line L92 (-21.318, -7.6564) -> (-21.318, -6.1555)
  line L93 (-21.318, -6.1555) -> (-21.5709, -6.1555)
  line L94 (-21.5709, -6.1555) -> (-21.5709, -7.6564)
  line L95 (-21.5709, -7.6564) -> (-21.318, -7.6564)
  line L96 (-2.3229, -4.083) -> (-2.3229, -3.2305)
  line L97 (-2.3229, -3.0198) -> (-2.3229, -2.8626)
  line L98 (-2.3229, -2.8626) -> (-2.5757, -2.8626)
  line L99 (-2.5757, -2.8626) -> (-2.5757, -4.9161)
  line L100 (-2.5757, -4.9161) -> (-2.3229, -4.9161)
  line L101 (-2.3229, -4.9161) -> (-2.3229, -4.2872)
  line L102 (-3.8432, -4.083) -> (-3.8432, -3.2305)
  line L103 (-3.8432, -3.0198) -> (-3.8432, -2.8626)
  line L104 (-3.8432, -2.8626) -> (-4.096, -2.8626)
  line L105 (-4.096, -2.8626) -> (-4.096, -4.9161)
  line L106 (-4.096, -4.9161) -> (-3.8432, -4.9161)
  line L107 (-3.8432, -4.9161) -> (-3.8432, -4.2872)
  line L108 (-4.4671, -4.3634) -> (-4.4671, -2.8626)
  line L109 (-4.4671, -2.8626) -> (-4.72, -2.8626)
  line L110 (-4.72, -2.8626) -> (-4.72, -4.3634)
  line L111 (-4.72, -4.3634) -> (-4.4671, -4.3634)
  line L112 (-5.707, -2.613) -> (-5.707, -2.3504)
  line L113 (-5.707, -2.3504) -> (-5.9939, -2.3504)
  line L114 (-5.9939, -2.3504) -> (-5.9939, -2.613)
  line L115 (-5.9939, -2.613) -> (-5.707, -2.613)
  line L116 (-6.2013, -2.6) -> (-6.2013, -2.3634)
  line L117 (-6.2013, -2.3634) -> (-7.3975, -2.3634)
  line L118 (-7.3975, -2.3634) -> (-7.3975, -4.3634)
  line L119 (-7.3975, -4.3634) -> (-7.1317, -4.3634)
  line L120 (-7.1317, -4.3634) -> (-7.1317, -3.4007)
  line L121 (-7.1317, -3.4007) -> (-6.2402, -3.4007)
  line L122 (-6.2402, -3.4007) -> (-6.2402, -3.1641)
  line L123 (-6.2402, -3.1641) -> (-7.1317, -3.1641)
  line L124 (-7.1317, -3.1641) -> (-7.1317, -2.6)
  line L125 (-7.1317, -2.6) -> (-6.2013, -2.6)
  line L126 (-8.647, -4.3634) -> (-8.647, -2.8626)
  line L127 (-8.647, -2.8626) -> (-8.8999, -2.8626)
  line L128 (-8.8999, -2.8626) -> (-8.8999, -4.3634)
  line L129 (-8.8999, -4.3634) -> (-8.647, -4.3634)
  line L130 (-10.1803, -4.3634) -> (-10.1803, -3.3893)
  line L131 (-11.1057, -3.0295) -> (-11.1057, -2.8626)
  line L132 (-11.1057, -2.8626) -> (-11.3586, -2.8626)
  line L133 (-11.3586, -2.8626) -> (-11.3586, -4.3634)
  line L134 (-11.3586, -4.3634) -> (-11.1057, -4.3634)
  line L135 (-11.1057, -4.3634) -> (-11.1057, -3.2418)
  line L136 (-10.4331, -3.5076) -> (-10.4331, -4.3634)
  line L137 (-10.4331, -4.3634) -> (-10.1803, -4.3634)
  line L138 (-11.861, -3.4461) -> (-12.6535, -3.4461)
  line L139 (-11.6422, -4.271) -> (-11.6422, -3.9955)
  line L140 (-11.6422, -3.9955) -> (-11.6568, -3.9955)
  line L141 (-12.6535, -3.6389) -> (-11.6146, -3.6389)
  line L142 (-11.6146, -3.6389) -> (-11.6146, -3.5012)
  line L143 (-16.9307, -4.3634) -> (-16.9307, -2.2743)
  line L144 (-16.9307, -2.2743) -> (-17.1835, -2.2743)
  line L145 (-17.1835, -2.2743) -> (-17.1835, -4.3634)
  line L146 (-17.1835, -4.3634) -> (-16.9307, -4.3634)
  line L147 (-17.7962, -3.5773) -> (-17.7962, -3.9939)
  line L148 (-17.7962, -4.2046) -> (-17.7962, -4.3634)
  line L149 (-17.7962, -4.3634) -> (-17.5433, -4.3634)
  line L150 (-17.5433, -4.3634) -> (-17.5433, -3.3375)
  line L151 (-18.6179, -2.895) -> (-18.6179, -3.1527)
  line L152 (-18.6179, -3.1527) -> (-18.6033, -3.1527)
  line L153 (-17.7962, -3.3277) -> (-17.7962, -3.3764)
  line L154 (-19.2516, -3.1316) -> (-19.2516, -3.9987)
  line L155 (-18.9987, -4.3634) -> (-18.9987, -2.2743)
  line L156 (-18.9987, -2.2743) -> (-19.2516, -2.2743)
  line L157 (-19.2516, -2.2743) -> (-19.2516, -2.9226)
  line L158 (-19.2516, -4.2111) -> (-19.2516, -4.3634)
  line L159 (-19.2516, -4.3634) -> (-18.9987, -4.3634)
  line L160 (-20.7605, -3.5773) -> (-20.7605, -3.9939)
  line L161 (-20.7605, -4.2046) -> (-20.7605, -4.3634)
  line L162 (-20.7605, -4.3634) -> (-20.5077, -4.3634)
  line L163 (-20.5077, -4.3634) -> (-20.5077, -3.3375)
  line L164 (-21.5822, -2.895) -> (-21.5822, -3.1527)
  line L165 (-21.5822, -3.1527) -> (-21.5676, -3.1527)
  line L166 (-20.7605, -3.3277) -> (-20.7605, -3.3764)
  line L167 (-3.3505, -0.1531) -> (-4.143, -0.1531)
  line L168 (-3.1317, -0.9781) -> (-3.1317, -0.7025)
  line L169 (-3.1317, -0.7025) -> (-3.1462, -0.7025)
  line L170 (-4.143, -0.346) -> (-3.1041, -0.346)
  line L171 (-3.1041, -0.346) -> (-3.1041, -0.2082)
  line L172 (-6.7378, -1.0705) -> (-6.7378, 0.4304)
  line L173 (-6.7378, 0.4304) -> (-6.9906, 0.4304)
  line L174 (-6.9906, 0.4304) -> (-6.9906, -0.6912)
  line L175 (-7.6633, -0.4254) -> (-7.6633, 0.4304)
  line L176 (-7.6633, 0.4304) -> (-7.9161, 0.4304)
  line L177 (-7.9161, 0.4304) -> (-7.9161, -0.5437)
  line L178 (-6.9906, -0.9051) -> (-6.9906, -1.0705)
  line L179 (-6.9906, -1.0705) -> (-6.7378, -1.0705)
  line L180 (-11.4898, -1.0705) -> (-11.237, -1.0705)
  line L181 (-11.237, -1.0705) -> (-11.237, -0.0818)
  line L182 (-12.9388, 0.265) -> (-12.9388, 0.4304)
  line L183 (-12.9388, 0.4304) -> (-13.1916, 0.4304)
  line L184 (-13.1916, 0.4304) -> (-13.1916, -1.0705)
  line L185 (-13.1916, -1.0705) -> (-12.9388, -1.0705)
  line L186 (-12.9388, -1.0705) -> (-12.9388, 0.0511)
  line L187 (-12.3407, -0.2017) -> (-12.3407, -1.0705)
  line L188 (-12.3407, -1.0705) -> (-12.0879, -1.0705)
  line L189 (-12.0879, -1.0705) -> (-12.0879, -0.0818)
  line L190 (-11.4898, -0.2017) -> (-11.4898, -1.0705)
  line L191 (-17.4412, -1.0705) -> (-17.4412, -0.0964)
  line L192 (-18.3667, 0.2634) -> (-18.3667, 0.4304)
  line L193 (-18.3667, 0.4304) -> (-18.6195, 0.4304)
  line L194 (-18.6195, 0.4304) -> (-18.6195, -1.0705)
  line L195 (-18.6195, -1.0705) -> (-18.3667, -1.0705)
  line L196 (-18.3667, -1.0705) -> (-18.3667, 0.0511)
  line L197 (-17.694, -0.2147) -> (-17.694, -1.0705)
  line L198 (-17.694, -1.0705) -> (-17.4412, -1.0705)
  line L199 (-19.2273, -0.2844) -> (-19.2273, -0.7009)
  line L200 (-19.2273, -0.9116) -> (-19.2273, -1.0705)
  line L201 (-19.2273, -1.0705) -> (-18.9744, -1.0705)
  line L202 (-18.9744, -1.0705) -> (-18.9744, -0.0445)
  line L203 (-20.049, 0.3979) -> (-20.049, 0.1402)
  line L204 (-20.049, 0.1402) -> (-20.0344, 0.1402)
  line L205 (-19.2273, -0.0348) -> (-19.2273, -0.0834)
  line L206 (-21.3099, -1.0705) -> (-21.3099, 1.0187)
  line L207 (-21.3099, 1.0187) -> (-21.5628, 1.0187)
  line L208 (-21.5628, 1.0187) -> (-21.5628, -1.0705)
  line L209 (-21.5628, -1.0705) -> (-21.3099, -1.0705)
  line L210 (-22.8902, -0.2844) -> (-22.5822, 0.6573)
  line L211 (-22.5822, 0.6573) -> (-22.2727, -0.2844)
  line L212 (-22.2727, -0.2844) -> (-22.8902, -0.2844)
  line L213 (-23.4137, -1.0705) -> (-23.1446, -1.0705)
  line L214 (-23.1446, -1.0705) -> (-22.9631, -0.5113)
  line L215 (-22.9631, -0.5113) -> (-22.1997, -0.5113)
  line L216 (-22.1997, -0.5113) -> (-22.0182, -1.0705)
  line L217 (-22.0182, -1.0705) -> (-21.7378, -1.0705)
  line L218 (-21.7378, -1.0705) -> (-22.412, 0.9295)
  line L219 (-22.412, 0.9295) -> (-22.7394, 0.9295)
  line L220 (-22.7394, 0.9295) -> (-23.4137, -1.0705)
  line L221 (-17.9987, 3.3408) -> (-17.9987, 3.7233)
  line L222 (-17.9987, 3.7233) -> (-18.3197, 3.7233)
  line L223 (-18.3197, 3.7233) -> (-18.3197, 3.3408)
  line L224 (-18.3197, 3.3408) -> (-17.9987, 3.3408)
  line L225 (-18.8156, 3.9729) -> (-18.8156, 4.2355)
  line L226 (-18.8156, 4.2355) -> (-19.1025, 4.2355)
  line L227 (-19.1025, 4.2355) -> (-19.1025, 3.9729)
  line L228 (-19.1025, 3.9729) -> (-18.8156, 3.9729)
  line L229 (-23.1106, 3.4526) -> (-23.1106, 3.7152)
  line L230 (-23.6535, 3.4996) -> (-23.6535, 3.7233)
  line L231 (-23.6535, 3.7233) -> (-23.9064, 3.7233)
  line L232 (-23.9064, 3.7233) -> (-23.9064, 2.2225)
  line L233 (-23.9064, 2.2225) -> (-23.6535, 2.2225)
  line L234 (-23.6535, 2.2225) -> (-23.6535, 3.2873)
  line L235 (-23.1235, 3.4526) -> (-23.1106, 3.4526)
  line L236 (-25.6697, 2.3068) -> (-25.6697, 2.5904)
  line L237 (-25.6697, 2.5904) -> (-25.6843, 2.5904)
  line L238 (-25.6843, 3.3586) -> (-25.6697, 3.3586)
  line L239 (-25.6697, 3.3586) -> (-25.6697, 3.6423)
  line L240 (-28.8902, 3.0086) -> (-28.5822, 3.9502)
  line L241 (-28.5822, 3.9502) -> (-28.2727, 3.0086)
  line L242 (-28.2727, 3.0086) -> (-28.8902, 3.0086)
  line L243 (-29.4137, 2.2225) -> (-29.1446, 2.2225)
  line L244 (-29.1446, 2.2225) -> (-28.9631, 2.7816)
  line L245 (-28.9631, 2.7816) -> (-28.1997, 2.7816)
  line L246 (-28.1997, 2.7816) -> (-28.0182, 2.2225)
  line L247 (-28.0182, 2.2225) -> (-27.7378, 2.2225)
  line L248 (-27.7378, 2.2225) -> (-28.412, 4.2225)
  line L249 (-28.412, 4.2225) -> (-28.7394, 4.2225)
  line L250 (-28.7394, 4.2225) -> (-29.4137, 2.2225)
  line L251 (1.5166, 6.7456) -> (1.5166, 7.0081)
  line L252 (0.9737, 6.7926) -> (0.9737, 7.0162)
  line L253 (0.9737, 7.0162) -> (0.7209, 7.0162)
  line L254 (0.7209, 7.0162) -> (0.7209, 5.5154)
  line L255 (0.7209, 5.5154) -> (0.9737, 5.5154)
  line L256 (0.9737, 5.5154) -> (0.9737, 6.5803)
  line L257 (1.5037, 6.7456) -> (1.5166, 6.7456)
  line L258 (-3.7929, 5.5154) -> (-3.5401, 5.5154)
  line L259 (-3.5401, 5.5154) -> (-3.5401, 6.5041)
  line L260 (-5.2419, 6.8509) -> (-5.2419, 7.0162)
  line L261 (-5.2419, 7.0162) -> (-5.4947, 7.0162)
  line L262 (-5.4947, 7.0162) -> (-5.4947, 5.5154)
  line L263 (-5.4947, 5.5154) -> (-5.2419, 5.5154)
  line L264 (-5.2419, 5.5154) -> (-5.2419, 6.637)
  line L265 (-4.6438, 6.3842) -> (-4.6438, 5.5154)
  line L266 (-4.6438, 5.5154) -> (-4.391, 5.5154)
  line L267 (-4.391, 5.5154) -> (-4.391, 6.5041)
  line L268 (-3.7929, 6.3842) -> (-3.7929, 5.5154)
  line L269 (-12.8075, 7.0162) -> (-13.0701, 7.0162)
  line L270 (-13.0701, 7.0162) -> (-13.4769, 5.8607)
  line L271 (-13.4769, 5.8607) -> (-13.8869, 7.0162)
  line L272 (-13.8869, 7.0162) -> (-14.1608, 7.0162)
  line L273 (-14.1608, 7.0162) -> (-13.6, 5.5154)
  line L274 (-13.6, 5.5154) -> (-13.3731, 5.5154)
  line L275 (-13.3731, 5.5154) -> (-12.8075, 7.0162)
  line L276 (-19.203, 7.2658) -> (-19.203, 7.5284)
  line L277 (-19.203, 7.5284) -> (-19.4898, 7.5284)
  line L278 (-19.4898, 7.5284) -> (-19.4898, 7.2658)
  line L279 (-19.4898, 7.2658) -> (-19.203, 7.2658)
  line L280 (-23.5806, 5.5997) -> (-23.5806, 5.8833)
  line L281 (-23.5806, 5.8833) -> (-23.5952, 5.8833)
  line L282 (-23.5952, 6.6516) -> (-23.5806, 6.6516)
  line L283 (-23.5806, 6.6516) -> (-23.5806, 6.9352)
  line L284 (-28.6308, 6.7034) -> (-28.9323, 6.7034)
  line L285 (-28.9323, 6.7034) -> (-28.9323, 7.2885)
  line L286 (-28.9323, 7.2885) -> (-28.6778, 7.2885)
  line L287 (-28.7167, 5.7423) -> (-28.9323, 5.7423)
  line L288 (-28.9323, 5.7423) -> (-28.9323, 6.4814)
  line L289 (-28.9323, 6.4814) -> (-28.6308, 6.4814)
  line L290 (-28.2159, 6.6273) -> (-28.2159, 6.637)
  line L291 (-28.6681, 7.5154) -> (-29.1981, 7.5154)
  line L292 (-29.1981, 7.5154) -> (-29.1981, 5.5154)
  line L293 (-29.1981, 5.5154) -> (-28.6244, 5.5154)
  line L294 (24.0742, 10.8975) -> (23.844, 10.8975)
  line L295 (23.844, 10.8975) -> (23.0645, 8.374)
  line L296 (23.0645, 8.374) -> (23.2914, 8.374)
  line L297 (23.2914, 8.374) -> (24.0742, 10.8975)
  line L298 (21.8732, 9.0547) -> (21.8602, 9.0547)
  line L299 (21.8602, 9.0547) -> (21.8602, 8.797)
  line L300 (18.4729, 8.8084) -> (18.4729, 9.0402)
  line L301 (18.4729, 9.0402) -> (17.4907, 9.0402)
  line L302 (17.2816, 10.7306) -> (17.2816, 10.4453)
  line L303 (17.2816, 10.4453) -> (17.2962, 10.4453)
  line L304 (17.2395, 9.092) -> (17.2395, 8.8084)
  line L305 (17.2395, 8.8084) -> (18.4729, 8.8084)
  line L306 (16.0466, 8.8084) -> (16.0466, 10.3092)
  line L307 (16.0466, 10.3092) -> (15.7938, 10.3092)
  line L308 (15.7938, 10.3092) -> (15.7938, 8.8084)
  line L309 (15.7938, 8.8084) -> (16.0466, 8.8084)
  line L310 (12.4097, 10.5588) -> (12.4097, 10.8214)
  line L311 (12.4097, 10.8214) -> (12.1228, 10.8214)
  line L312 (12.1228, 10.8214) -> (12.1228, 10.5588)
  line L313 (12.1228, 10.5588) -> (12.4097, 10.5588)
  line L314 (11.8975, 8.8084) -> (11.8975, 9.0207)
  line L315 (11.8975, 9.0207) -> (11.0953, 9.0207)
  line L316 (11.0953, 9.0207) -> (11.8829, 10.1293)
  line L317 (11.8829, 10.1293) -> (11.8829, 10.3092)
  line L318 (11.8829, 10.3092) -> (10.8278, 10.3092)
  line L319 (10.8278, 10.3092) -> (10.8278, 10.1017)
  line L320 (10.8278, 10.1017) -> (11.5799, 10.1017)
  line L321 (11.5799, 10.1017) -> (10.7954, 8.9964)
  line L322 (10.7954, 8.9964) -> (10.7954, 8.8084)
  line L323 (10.7954, 8.8084) -> (11.8975, 8.8084)
  line L324 (10.3043, 9.5944) -> (10.3043, 9.1779)
  line L325 (10.3043, 8.9672) -> (10.3043, 8.8084)
  line L326 (10.3043, 8.8084) -> (10.5572, 8.8084)
  line L327 (10.5572, 8.8084) -> (10.5572, 9.8343)
  line L328 (9.4826, 10.2768) -> (9.4826, 10.0191)
  line L329 (9.4826, 10.0191) -> (9.4972, 10.0191)
  line L330 (10.3043, 9.844) -> (10.3043, 9.7954)
  line L331 (6.6025, 10.5588) -> (6.6025, 10.8214)
  line L332 (6.6025, 10.8214) -> (6.3157, 10.8214)
  line L333 (6.3157, 10.8214) -> (6.3157, 10.5588)
  line L334 (6.3157, 10.5588) -> (6.6025, 10.5588)
  line L335 (6.1358, 10.3092) -> (5.8732, 10.3092)
  line L336 (5.8732, 10.3092) -> (5.4664, 9.1536)
  line L337 (5.4664, 9.1536) -> (5.0564, 10.3092)
  line L338 (5.0564, 10.3092) -> (4.7825, 10.3092)
  line L339 (4.7825, 10.3092) -> (5.3432, 8.8084)
  line L340 (5.3432, 8.8084) -> (5.5701, 8.8084)
  line L341 (5.5701, 8.8084) -> (6.1358, 10.3092)
  line L342 (3.5961, 9.7257) -> (2.8035, 9.7257)
  line L343 (3.8149, 8.9008) -> (3.8149, 9.1763)
  line L344 (3.8149, 9.1763) -> (3.8003, 9.1763)
  line L345 (2.8035, 9.5329) -> (3.8424, 9.5329)
  line L346 (3.8424, 9.5329) -> (3.8424, 9.6706)
  line L347 (1.6512, 8.8084) -> (1.6512, 10.8975)